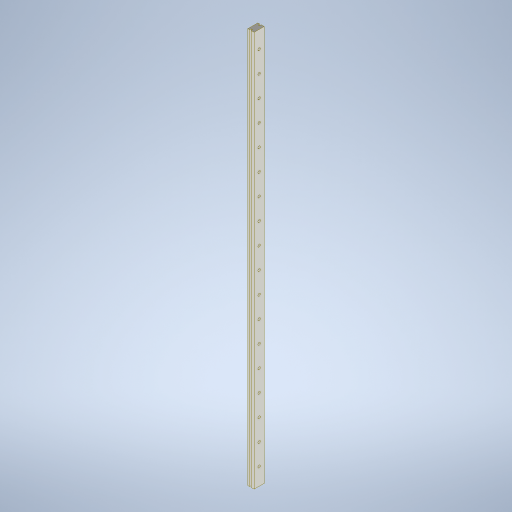
# Autodesk Inventor part: Trilho 2
Saved by Autodesk Inventor 2023.2 (Build 272271030, 271C)
## iProperties
Created: 2023-04-01
Part Number: Trilho 2
Material: Aço inoxidável
Document SubType Name: Sheet Metal
Designer: Mateus PC
Density: 8 g/cm^3
Sheet Metal Rule: Padrão_mm
Appearance: Prata
Author: Mateus PC
Autodesk Inventor part; units mm, degrees
ref_plane "YZ Plane" through (0, 0, 0) normal (1, 0, 0) x (0, 1, 0)
ref_plane "XZ Plane" through (0, 0, 0) normal (0, 1, 0) x (-1, 0, 0)
ref_plane "XY Plane" through (0, 0, 0) normal (0, 0, 1) x (1, 0, 0)
sketch "Esboço1" plane through (0, 0, 0) normal (0, 1, 0) x (-1, 0, 0)
  line L0 (0, 0) -> (3.5, 0)
  line L1 (4, -2) -> (5, -2)
  line L2 (5.5, 0) -> (7.5, 0)
  line L3 (7.5, 0) -> (7.5, -12)
  line L4 (7.5, -12) -> (5.5, -12)
  line L5 (5, -10) -> (4, -10)
  line L6 (3.5, -12) -> (0, -12)
  line L7 (0, -12) -> (0, 0)
  line L8 (5.5, 0) -> (5, -2)
  line L9 (3.5, 0) -> (4, -2)
  line L10 (5, -10) -> (5.5, -12)
  line L11 (3.5, -12) -> (4, -10)
  dimension "d0" = 7.5
  dimension "d1" = 12
  dimension "d2" = 8
  dimension "d3" = 1
  dimension "d4" = 3.5
  dimension "d5" = 0.5
  constraints: 24 end point, 4 point on line, 3 equal length, 3 perpendicular, 1 horizontal, 1 parallel
  measures "d0" distance of L0.start L2.end
  measures "d1" distance of L6.end L0.start
  measures "d2" distance of L1.end L5.start
  measures "d3" distance of L1.start L1.end
  measures "d4" distance of L0.start L0.end
  measures "d5" horizontal distance of L2.start L1.end
extrude "Extrusão1" add sketch "Esboço1" along normal blind 469
sketch "Esboço2" plane through (-7.5, 0, -12) normal (-1, 0, 0) x (0, 0, 1)
  line L0 (0, 0) -> (0, 469) projected
  line L1 (0, 0) -> (12, 0) projected
  line L2 (12, 0) -> (12, 469) projected
  point P0 (6, 20.3)
  point P1 (6, 45.5)
  point P2 (6, 70.7)
  point P3 (6, 95.9)
  point P4 (6, 121.1)
  point P5 (6, 146.3)
  point P6 (6, 171.5)
  point P7 (6, 196.7)
  point P8 (6, 221.9)
  point P9 (6, 247.1)
  point P10 (6, 272.3)
  point P11 (6, 297.5)
  point P12 (6, 322.7)
  point P13 (6, 347.9)
  point P14 (6, 373.1)
  point P15 (6, 398.3)
  point P16 (6, 423.5)
  point P17 (6, 448.7)
  point P18 (6, 0)
  point P19 (6, 473.9)
  dimension "d10" = 25.2
  dimension "d15" = 428.4
  dimension "d16" = 469
  dimension "d17" = 20.3
  dimension "d18" = 6
  constraints: 1 midpoint, 1 vertical, 18 other
  measures "d10" distance of point (6, 20.3) point (6, 45.5)
  measures "d15" distance of point (6, 448.7) point (6, 20.3)
  measures "d16" distance of L0.start L0.end
  measures "d17" distance of point (6, 0) point (6, 20.3)
  measures "d18" distance from line of L2 point (6, 20.3)
hole "Furo1" at (-7.5, 20.3, -6) at (-7.5, 45.5, -6) at (-7.5, 70.7, -6) at (-7.5, 95.9, -6) at (-7.5, 121.1, -6) at (-7.5, 146.3, -6) at (-7.5, 171.5, -6) at (-7.5, 196.7, -6) at (-7.5, 221.9, -6) at (-7.5, 247.1, -6) at (-7.5, 272.3, -6) at (-7.5, 297.5, -6) at (-7.5, 322.7, -6) at (-7.5, 347.9, -6) at (-7.5, 373.1, -6) at (-7.5, 398.3, -6) at (-7.5, 423.5, -6) at (-7.5, 448.7, -6) direction (1, 0, 0) diameter 3 depth 7.5 tip angle 118 counterbore diameter 4 counterbore depth 2
equation "\"d17\" = -0.5 * d15 + 0.5 * d16"
equation "\"d24\" = Espessura"
equation "\"Raio_vergadura\" = Espessura"
equation "\"Largura_alívio_de_vergadura\" = Espessura"
equation "\"Profundidade_alívio_de_vergadura\" = 0.5 * Espessura"
equation "\"Tamanho_alívio_de_dobra\" = 4 * Espessura"
equation "\"Remanescente_mínimo\" = 2 * Espessura"
equation "\"Raiodetransição\" = Raio_vergadura"
equation "\"Tamanho_de_raio_de_Jacobi\" = Raio_vergadura"
equation "\"TamanhoFolga\" = Espessura"
equation "\"Espessura\" = 0.5"
